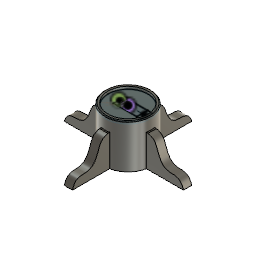
Base (Autodesk Fusion 360 design; units mm, degrees)
part number: 2026-08-14-15-29-28-513
Autodesk Fusion 360 part; units mm, degrees
sketch "Sketch1" plane through (0, 0, 0) normal (0, 0, 1) x (1, 0, 0)
  circle A0 centre (0, 0) radius 27.5
  dimension "d1" = 55
  constraint coincident A0.centre origin
  measures "d1" diameter of A0
extrude "Extrude1" add sketch "Sketch1" along normal blind 50
sketch "Sketch2" plane through (0, 0, 0) normal (0, 1, 0) x (1, 0, 0)
  line L0 (29, -50) -> (29, -37.898) construction
  line L1 (29, 0) -> (71.7823, 0)
  spline S0 degree 5 poles (29, -37.898) (29.3615, -37.8796) (30.0907, -37.8033) (31.2034, -37.5708) (32.7047, -37.0332) (34.5058, -36.029) (36.1177, -34.7441) (37.4625, -33.2157) (38.5477, -31.4446) (39.4457, -29.415) (40.2655, -27.1187) (41.1293, -24.5767) (42.1453, -21.8656) (43.3866, -19.1327) (44.8964, -16.5569) (46.6897, -14.3184) (48.7553, -12.5626) (51.0579, -11.3701) (53.5391, -10.714) (56.1219, -10.4581) (58.7202, -10.4029) (61.2479, -10.3181) (63.6265, -9.9787) (65.7954, -9.2037) (67.7174, -7.8813) (69.3719, -5.9478) (70.4746, -3.8904) (71.1769, -2.0576) (71.5897, -0.7073) (71.7823, 0) knots 0 0 0 0 0 0 0.04 0.08 0.12 0.16 0.2 0.24 0.28 0.32 0.36 0.4 0.44 0.48 0.52 0.56 0.6 0.64 0.68 0.72 0.76 0.8 0.84 0.88 0.92 0.96 1 1 1 1 1 1
  line L2 (29, -37.898) -> (27, -38)
  line L3 (27, -38) -> (26.7815, 0)
  line L4 (26.7815, 0) -> (29, 0)
  point P0 (36.1963, -34.5428)
  point P1 (41, -25)
  point P2 (50, -12)
  point P3 (63, -10)
  dimension "d7" = 45
  constraint vertical L0
  measures "d7" distance of L1.end L3
extrude "Extrude2" add sketch "Sketch2" along normal mid plane 10
pattern_circular "C-Pattern1" count 4 over 360 about axis through (0, 0, 50) along (0, 0, 1) of "Extrude2"
sketch "Sketch3" plane through (0, 0, 50) normal (0, 0, 1) x (-1, 0, 0)
  circle A0 centre (0, 0) radius 27.5
  circle A1 centre (0, 0) radius 3.15
  line L0 (-17.1, -6.5) -> (11, -6.5)
  line L1 (11, -6.5) -> (11, 6.5)
  line L2 (11, 6.5) -> (-17.1, 6.5)
  line L3 (-17.1, 6.5) -> (-17.1, -6.5)
  line L4 (6.1, -6.5) -> (6.1, 6.5)
  line L5 (-17.1, 6.5) -> (-22, 6.5)
  line L6 (-22, 6.5) -> (-22, -6.5)
  line L7 (-22, -6.5) -> (-17.1, -6.5)
  line L8 (-22, 0) -> (11, 0) construction
  line L9 (6.1, -6.5) -> (11, 6.5) construction
  line L10 (6.1, 6.5) -> (11, -6.5) construction
  circle A2 centre (8.55, 0) radius 1
  line L11 (-22, -6.5) -> (-17.1, 6.5) construction
  line L12 (-22, 6.5) -> (-17.1, -6.5) construction
  circle A3 centre (-19.55, 0) radius 1
  circle A4 centre (0, 0) radius 24
  dimension "d10" = 6.3
  dimension "d11" = 11
  dimension "d12" = 4.9
  dimension "d13" = 23.2
  dimension "d14" = 4.9
  dimension "d16" = 13
  dimension "d19" = 2
  dimension "d20" = 2
  dimension "d23" = -3.5
  constraint coincident A0.centre A1.centre
  constraint horizontal L0
  constraint vertical L1
  constraint horizontal L2
  constraint vertical L3
  constraint coincident L0 L4.start
  constraint coincident L2 L4.end
  constraint perpendicular L2 L4
  constraint perpendicular L3 L5
  constraint perpendicular L5 L6
  constraint perpendicular L3 L7
  constraint midpoint L6 L8.start
  constraint midpoint L1 L8.end
  constraint midpoint L10 A2.centre
  constraint midpoint L12 A3.centre
  measures "d10" diameter of A1
  measures "d11" distance of A0.centre L1
  measures "d12" distance of L1 L4
  measures "d13" distance of L3 L4
  measures "d14" distance of L3 L6
  measures "d16" distance of L0.end L1.end
  measures "d19" diameter of A2
  measures "d20" diameter of A3
extrude "Extrude3" cut sketch "Sketch3" against normal blind 17 contours A1 | L0 L2 L3 L4
extrude "Extrude4" cut sketch "Sketch3" against normal blind 10 contours A2 | A3
extrude "Extrude5" add sketch "Sketch3" along normal blind 3 contours A0
fillet "Fillet1" radius 1 1 edges at (25.639, 9.9444, 53)
sketch "Sketch4" plane through (-6.1, 0, 0) normal (1, 0, 0) x (0, 1, 0)
  line L0 (6.5, 50) -> (-6.5, 50)
  line L1 (-6.5, 50) -> (-6.5, 33)
  line L2 (-6.5, 33) -> (6.5, 33)
  line L3 (6.5, 33) -> (6.5, 50)
  line L4 (-6.5, 50) -> (6.5, 50) construction
  line L5 (6.5, 50) -> (6.5, 33) construction
  line L6 (6.5, 33) -> (-6.5, 33) construction
  line L7 (-6.5, 33) -> (-6.5, 50) construction
  line L8 (2.5, 47.5) -> (-2.5, 47.5)
  line L9 (-2.5, 47.5) -> (-2.5, 35.5)
  line L10 (-2.5, 35.5) -> (2.5, 35.5)
  line L11 (2.5, 35.5) -> (2.5, 47.5)
  line L12 (2.5, 47.5) -> (-2.5, 35.5) construction
  line L13 (-2.5, 47.5) -> (2.5, 35.5) construction
  point P0 (0, 41.5)
  dimension "d28" = 5
  dimension "d29" = 12
  dimension "d30" = 2.5
  constraint horizontal L4
  constraint vertical L5
  constraint horizontal L6
  constraint vertical L7
  constraint coincident L2.end L3.start
  constraint coincident L0.end L1.start
  constraint horizontal L8
  constraint perpendicular L8 L9
  constraint parallel L8 L10
  constraint parallel L9 L11
  constraint coincident L12 P0
  constraint coincident L13 P0
  measures "d28" distance of L8.start L8.end
  measures "d30" distance of L6 L10
extrude "Extrude6" cut sketch "Sketch4" against normal blind 22 contours L8 L9 L10 L11
